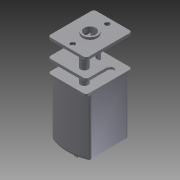
# Autodesk Inventor part: launcher.motor.main
Saved by Autodesk Inventor 2011 (Build 150239000, 239)
## iProperties
Created: 2011-04-05
Part Number: launcher.motor.main
Document SubType Name: Modeling
Designer: Rob
Density: 1 g/cm^3
Author: Rob
Autodesk Inventor part; units mm, degrees
note: some values were not read from the file. Chosen so that the rebuilt part matches the saved one: direction of "Hole1".
sketch "Sketch1" plane through (0, 0, 0) normal (0, 0, 1) x (1, 0, 0)
  line L0 (-5, 6) -> (5, 6)
  line L1 (5, 6) -> (5, -6)
  line L2 (5, -6) -> (-5, -6)
  line L3 (-5, -6) -> (-5, 6)
  line L4 (0, 0) -> (0, 26.0828)
  line L5 (0, 0) -> (22.7623, 0)
  line L6 (5, -4.9004) -> (-5, -4.9004)
  arc A0 (-5, -4.9004) -> (5, -4.9004) centre (0, 6) ccw
  arc A1 (5, 4.9004) -> (-5, 4.9004) centre (0, -6) ccw
  line L7 (5, -4.9004) -> (5, 4.9004)
  line L8 (-5, -4.9004) -> (-5, 4.9004)
  line L9 (5, 4.9004) -> (5, 6)
  line L10 (5, 6) -> (-5, 6)
  line L11 (-5, 4.9004) -> (-5, 6)
  dimension "d0" = 10
  dimension "d1" = 12
  constraints: 24 end point, 4 collinear, 4 perpendicular, 4 point on circle, 3 parallel, 3 symmetric about line, 2 centre point, 2 point on line, 1 horizontal, 1 midpoint, 3 other
  measures "d0" distance of L1.end L2.end
  measures "d1" distance of L0.end L1.end
ref_plane "Work Plane2" through (0, 0, 0) normal (0, 0, -1) x (-1, 0, 0)
extrude "Extrusion4" add sketch "Sketch1" along normal blind 15 contours A1 L4 L5 L1 L6 L3 | A1 L1 L5 L4 | L6 A0
sketch "Sketch4" plane through (0, 0, 0) normal (0, 0, -1) x (-1, 0, 0)
  circle A0 centre (0, 0) radius 2.5
  line L0 (0.5, -3.65) -> (-0.5, -3.65)
  line L1 (-0.5, -3.65) -> (-0.5, -3.35)
  line L2 (-0.5, -3.35) -> (0.5, -3.35)
  line L3 (0.5, -3.35) -> (0.5, -3.65)
  line L4 (0.5, 3.35) -> (-0.5, 3.35)
  line L5 (-0.5, 3.35) -> (-0.5, 3.65)
  line L6 (-0.5, 3.65) -> (0.5, 3.65)
  line L7 (0.5, 3.65) -> (0.5, 3.35)
  line L8 (0, 0) -> (0, -1.0426)
  line L9 (0.5, -3.5) -> (-0.5, -3.5)
  line L10 (-0.5, 3.5) -> (0.5, 3.5)
  line L11 (0, 0) -> (-0.9249, 0)
  dimension "d20" = 5
  dimension "d21" = 1
  dimension "d22" = 0.3
  dimension "d23" = 1
  dimension "d24" = 0.3
  dimension "d25" = 7
  constraints: 24 end point, 6 parallel, 4 midpoint, 4 perpendicular, 2 horizontal, 1 centre point, 1 coincident, 1 collinear, 4 other
  measures "d20" diameter of A0
  measures "d21" distance of L1.end L2.end
  measures "d22" distance of L0.end L1.end
  measures "d23" distance of L5.end L6.end
  measures "d24" distance of L4.end L5.end
  measures "d25" distance between parallel lines of L10 L9
extrude "Extrusion5" add sketch "Sketch4" along normal blind 2
fillet "Fillet2" radius 0.7 8 edges at (-5, -4.9004, 7.5) (-5, 4.9004, 7.5) (5, 4.9004, 7.5) (5, -4.9004, 7.5) (0, -5.9924, 0) (5, 0, 0) (-5, 0, 0) (0, 5.9924, 0)
ref_plane "Work Plane3" through (0, 0, 24) normal (0, 0, 1) x (1, 0, 0)
sketch "Sketch5" plane through (0, 0, 15) normal (0, 0, 1) x (1, 0, 0)
  line L0 (5, -6) -> (-5, -6)
  line L1 (-5, -6) -> (-5, 6)
  line L2 (-5, 6) -> (5, 6)
  line L3 (5, 6) -> (5, -6)
  line L4 (0, 0) -> (0, -2.6085)
  line L5 (0, 0) -> (2.5833, 0)
  dimension "d30" = 10
  dimension "d31" = 12
  constraints: 12 end point, 3 parallel, 2 perpendicular, 1 horizontal, 2 other
  measures "d30" distance of L1.end L2.end
  measures "d31" distance of L2.end L0.start
extrude "Extrusion6" add sketch "Sketch5" along normal blind 0.7
fillet "Fillet3" radius 0.7 4 edges at (-5, -6, 15.35) (-5, 6, 15.35) (5, 6, 15.35) (5, -6, 15.35)
sketch "Sketch6" plane through (0, 0, 24) normal (0, 0, 1) x (1, 0, 0)
  line L0 (5, -6) -> (-5, -6)
  line L1 (-5, -6) -> (-5, 6)
  line L2 (-5, 6) -> (5, 6)
  line L3 (5, 6) -> (5, -6)
  line L4 (0, 0) -> (-2.364, 0)
  line L5 (0, 0) -> (0, -2.8758)
  dimension "d35" = 10
  dimension "d36" = 12
  constraints: 12 end point, 3 perpendicular, 2 parallel, 1 horizontal, 2 other
  measures "d35" distance of L1.end L2.end
  measures "d36" distance of L0.end L1.end
extrude "Extrusion7" add sketch "Sketch6" against normal blind 0.7
fillet "Fillet4" radius 0.7 4 edges at (-5, -6, 23.65) (5, -6, 23.65) (-5, 6, 23.65) (5, 6, 23.65)
sketch "Sketch7" plane through (0, 0, 15.7) normal (0, 0, 1) x (1, 0, 0)
  line L0 (4.3, -6) -> (-4.3, -6) projected
  line L1 (-3.7781, 4.5) -> (3.9828, 4.5)
  line L2 (-3.5521, -4.5) -> (3.9209, -4.5)
  line L3 (0, 0) -> (2.1479, 0)
  line L4 (0, 0) -> (0, -1.7854)
  line L5 (-2.0293, 4.5) -> (-2.0293, 2.4975)
  line L6 (2.0293, -4.5) -> (2.0293, -2.5)
  circle A0 centre (-2.0293, 3.5) radius 1
  circle A1 centre (2.0293, -3.5) radius 1
  dimension "d40" = 2
  dimension "d42" = 2
  dimension "d41" = 4.5
  constraints: 12 end point, 4 parallel, 3 point on line, 2 perpendicular, 2 vertical alignment, 1 midpoint, 6 other
  measures "d41" distance between parallel lines of L1 L3
extrude "Extrusion8" add sketch "Sketch7" along normal up to surface (7.6 mm away)
sketch "Sketch8" plane through (0, 0, 24) normal (0, 0, 1) x (1, 0, 0)
  circle A0 centre (0, 0) radius 1.95
  dimension "d45" = 3.9
  constraints: 1 centre point, 1 coincident
  measures "d45" diameter of A0
extrude "Extrusion9" add sketch "Sketch8" along normal blind 0.6
sketch "Sketch10" plane through (0, 0, 24.6) normal (0, 0, 1) x (1, 0, 0)
  circle A0 centre (0, 0) radius 1.95 projected
  circle A1 centre (0, 0) radius 1.5
  dimension "d52" = 3
  constraints: 1 centre point, 1 coincident
  measures "d52" diameter of A1
extrude "Extrusion11" cut sketch "Sketch10" against normal blind 5.67 contours A1
ref_plane "Work Plane4" through (0, 0, 19.2) normal (0, 0, 1) x (1, 0, 0)
sketch "Sketch11" plane through (0, 0, 19.2) normal (0, 0, 1) x (1, 0, 0)
  line L0 (-5, 6) -> (0, 6)
  line L1 (0, 6) -> (0, -6)
  line L2 (0, -6) -> (-5, -6)
  line L3 (-5, -6) -> (-5, 6)
  line L4 (0, 0) -> (0, -2.3516)
  line L5 (0, 0) -> (-2.2311, 0)
  line L6 (-5, -6) -> (5, -6)
  line L7 (5, -6) -> (5, 0)
  line L8 (5, 0) -> (-5, 0)
  line L9 (-5, 0) -> (-5, -6)
  line L10 (0, 1.4288) -> (1.4337, 0)
  line L11 (0, 1.4288) -> (0, 0)
  line L12 (0, 0) -> (1.4337, 0)
  dimension "d56" = 5
  dimension "d57" = 12
  dimension "d58" = 10
  constraints: 26 end point, 5 parallel, 3 perpendicular, 2 collinear, 2 horizontal, 2 point on line, 1 other
  measures "d56" distance of L1.end L2.end
  measures "d57" distance of L0.end L1.end
  measures "d58" distance of L8.end L7.end
extrude "Extrusion12" add sketch "Sketch11" against normal blind 0.7
sketch "Sketch12" plane through (0, 0, 15.7) normal (0, 0, 1) x (1, 0, 0)
  line L0 (5, 5.3) -> (5, -5.3) projected
  line L1 (-4.3, 6) -> (4.3, 6) projected
  circle A0 centre (2.5, 3) radius 0.75
  point P0 (0, 0)
  dimension "d62" = 1.5
  dimension "d63" = 2.5
  dimension "d64" = 3
  constraints: 1 centre point
  measures "d62" diameter of A0
  measures "d63" distance from line of L0 A0.centre
  measures "d64" distance from line of A0.centre L1
extrude "Extrusion13" cut sketch "Sketch12" against normal blind 0.5
fillet "Fillet6" radius 0.7 7 edges at (0, 1.4288, 18.85) (1.4337, 0, 18.85) (5, 0, 18.85) (0, 6, 18.85) (-5, 6, 18.85) (-5, -6, 18.85) (5, -6, 18.85)
sketch "Sketch13" plane through (0, 0, 23.3) normal (0, 0, -1) x (-1, 0, 0)
  line L0 (-5, -5.3) -> (-5, 5.3) projected
  line L1 (-4.3, 6) -> (4.3, 6) projected
  circle A0 centre (-2.5, 3) radius 0.75
  dimension "d68" = 1.5
  dimension "d69" = 3
  dimension "d70" = 2.5
  constraints: 1 centre point
  measures "d68" diameter of A0
  measures "d69" distance from line of A0.centre L1
  measures "d70" distance from line of L0 A0.centre
extrude "Extrusion14" cut sketch "Sketch13" against normal blind 0.3
sketch "Sketch14" plane through (0, 0, 19.2) normal (0, 0, 1) x (1, 0, 0)
  circle A0 centre (0, 0) radius 0.5
  dimension "d73" = 1
  constraints: 1 centre point, 1 coincident
  measures "d73" diameter of A0
extrude "Extrusion15" cut sketch "Sketch14" against normal blind 0.3
sketch "Sketch15" plane through (0, 0, 24) normal (0, 0, 1) x (1, 0, 0)
  circle A0 centre (0, 0) radius 1.95 projected
  circle A1 centre (0, -4.5) radius 0.75
  circle A2 centre (0, 4.5) radius 0.75
  dimension "d76" = 1.5
  dimension "d77" = 1.5
  dimension "d78" = 4.5
  dimension "d79" = 4.5
  constraints: 2 centre point
  measures "d76" diameter of A1
  measures "d77" diameter of A2
  measures "d78" distance of A1.centre A0.centre
  measures "d79" distance of A2.centre A0.centre
hole "Hole1" at (0, -4.5, 24) at (0, 4.5, 24) direction (0, 0, -1) diameter 1.221 end up to surface thread size "M1.6x0.35" class "6H" standard "ANSI Metric M Profile"
body "Solid1"
